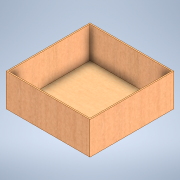
# Autodesk Inventor part: Gabarito
Saved by Autodesk Inventor 2021 (Build 250183000, 183)
## iProperties
Created: 2022-10-20
Part Number: Gabarito
Material: Madeira (Cerejeira)
Document SubType Name: Modeling
Designer: nicho
Appearance: Cerejeira - Natural com pouco brilho
Surface Area: 530.98 cm^2
Volume: 39.36 cm^3
Author: nicho
Autodesk Inventor part; units mm, degrees
ref_plane "YZ Plane" through (0, 0, 0) normal (1, 0, 0) x (0, 1, 0)
ref_plane "XZ Plane" through (0, 0, 0) normal (0, 1, 0) x (-1, 0, 0)
ref_plane "XY Plane" through (0, 0, 0) normal (0, 0, 1) x (1, 0, 0)
sketch "Esboço1" plane through (0, 0, 0) normal (0, 1, 0) x (-1, 0, 0)
  line L0 (-51.5, 51.5) -> (51.5, 51.5)
  line L1 (51.5, 51.5) -> (51.5, -51.5)
  line L2 (51.5, -51.5) -> (-51.5, -51.5)
  line L3 (-51.5, -51.5) -> (-51.5, 51.5)
  line L4 (-51.5, 51.5) -> (51.5, -51.5) construction
  line L5 (51.5, 51.5) -> (-51.5, -51.5) construction
  point P0 (0, 0)
  dimension "d0" = 103
  dimension "d1" = 103
  constraints: 12 end point, 2 midpoint, 2 parallel, 1 horizontal, 1 perpendicular
  measures "d0" distance of L1.end L2.end
  measures "d1" distance of L0.end L1.end
extrude "Extrusão1" add sketch "Esboço1" along normal blind 40
sketch "Esboço2" plane through (0, 40, 0) normal (0, 1, 0) x (1, 0, 0)
  line L0 (51.5, 51.5) -> (-51.5, 51.5) projected
  line L1 (-51.5, 51.5) -> (-51.5, -51.5) projected
  line L2 (-51.5, -51.5) -> (51.5, -51.5) projected
  line L3 (51.5, -51.5) -> (51.5, 51.5) projected
  line L4 (-50, -50) -> (-50, 50)
  line L5 (-50, 50) -> (50, 50)
  line L6 (50, 50) -> (50, -50)
  line L7 (50, -50) -> (-50, -50)
  point P0 (0, 0)
  dimension "d4" = 1.5
  constraints: 8 end point, 3 other
  measures "d4" distance between parallel lines of L1 L4
extrude "Extrusão2" cut sketch "Esboço2" against normal blind 38.5 contours L4 L5 L6 L7
